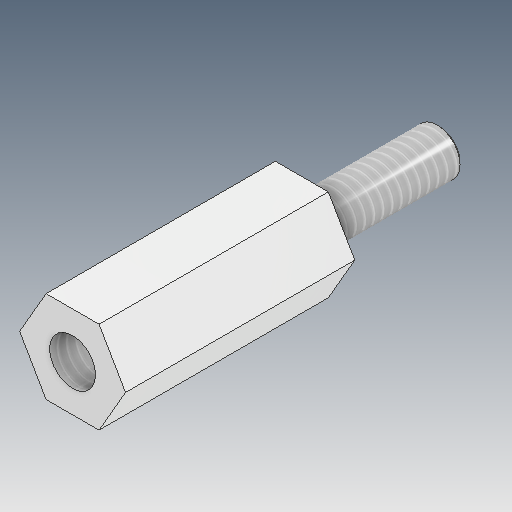
# Autodesk Inventor part: Espaciador de Plástico M2 L10
Saved by Autodesk Inventor 2020 (Build 240168000, 168)
## iProperties
Created: 2020-08-20
Part Number: Espaciador de Plástico M2 L10
Material: Brass, Soft Yellow
Document SubType Name: Modeling
Designer: Dante
Density: 8.47 g/cm^3
Appearance: PVC - White
Author: Dante
Autodesk Inventor part; units mm, degrees
ref_plane "YZ Plane" through (0, 0, 0) normal (1, 0, 0) x (0, 1, 0)
ref_plane "XZ Plane" through (0, 0, 0) normal (0, 1, 0) x (-1, 0, 0)
ref_plane "XY Plane" through (0, 0, 0) normal (0, 0, 1) x (1, 0, 0)
sketch "Sketch1" plane through (0, 0, 0) normal (0, 0, 1) x (1, 0, 0)
  line L0 (-7.5896, 2.5423) -> (-6.4349, 4.5423)
  line L1 (-6.4349, 4.5423) -> (-4.1255, 4.5423)
  line L2 (-4.1255, 4.5423) -> (-2.9708, 2.5423)
  line L3 (-2.9708, 2.5423) -> (-4.1255, 0.5423)
  line L4 (-4.1255, 0.5423) -> (-6.4349, 0.5423)
  line L5 (-6.4349, 0.5423) -> (-7.5896, 2.5423)
  circle A0 centre (-5.2802, 2.5423) radius 1
  dimension "d0" = 4
  dimension "d1" = 2
  constraints: 12 end point, 1 centre point, 1 coincident, 13 other
  measures "d0" distance between parallel lines of L4 L1
  measures "d1" diameter of A0
extrude "Extrusion1" add sketch "Sketch1" along normal blind 10 contours L0 L1 L2 L3 L4 L5 | A0
extrude "Extrusion2" add sketch "Sketch1" against normal blind 6 contours A0
sketch "Sketch2" plane through (0, 0, 10) normal (0, 0, 1) x (1, 0, 0)
  circle A0 centre (-5.2802, 2.5423) radius 1 projected
  circle A1 centre (-5.2802, 2.5423) radius 1.5
  point P0 (0, 0)
  constraints: 1 centre point, 1 coincident
hole "Hole1" at (-5.2802, 2.5423, 10) direction (0, 0, -1) diameter 2 depth 7 tip angle 120
chamfer "Chamfer1" distance 0.1 angle 45 1 edges at (-6.2802, 2.5423, -6)
thread "Thread3" size "M2x0.4" class "6g" standard "ISO Metric profile" length 6
thread "Thread4" size "M2x0.4" class "6H" standard "ISO Metric profile" length 6
body "Solid1"
